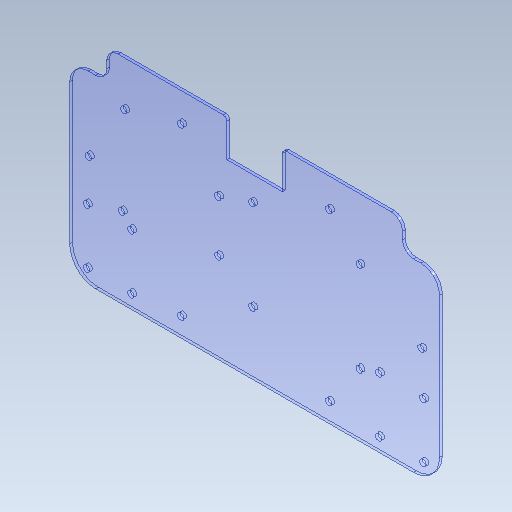
# Autodesk Inventor part: upper_frame
Saved by Autodesk Inventor 2020 (Build 240168000, 168)
## iProperties
Created: 2020-06-24
Part Number: upper_frame
Material: アルミニウム 6061
Document SubType Name: Modeling
Designer: haya
Density: 2.7 g/cm^3
Appearance: クリア - 青
Author: haya
Autodesk Inventor part; units mm, degrees
ref_plane "YZ Plane" through (0, 0, 0) normal (1, 0, 0) x (0, 1, 0)
ref_plane "XZ Plane" through (0, 0, 0) normal (0, 1, 0) x (-1, 0, 0)
ref_plane "XY Plane" through (0, 0, 0) normal (0, 0, 1) x (1, 0, 0)
sketch "スケッチ1" plane through (0, 0, 0) normal (0, 0, 1) x (1, 0, 0)
  line L0 (0, 0) -> (200, 0)
  line L1 (200, 0) -> (200, 100)
  line L2 (200, 100) -> (0, 100)
  line L3 (0, 100) -> (0, 0)
  dimension "d2" = 200
  dimension "d3" = 100
  constraints: 8 end point, 2 parallel, 1 horizontal, 1 perpendicular
  measures "d2" distance of L0.start L0.end
  measures "d3" distance of L2.end L0.start
extrude "押し出し1" add sketch "スケッチ1" along normal blind 1.5
fillet "フィレット1" radius 10 2 edges at (0, 100, 0.75) (200, 100, 0.75)
fillet "フィレット2" radius 14 2 edges at (200, 0, 0.75) (0, 0, 0.75)
sketch "スケッチ2" plane through (0, 0, 0) normal (0, 0, -1) x (-1, 0, 0)
  line L0 (-190, 100) -> (-10, 100) projected
  line L1 (-180, 100) -> (-20, 100)
  line L2 (-20, 100) -> (-20, 116)
  line L3 (-20, 116) -> (-180, 116)
  line L4 (-180, 116) -> (-180, 100)
  line L5 (0, 90) -> (0, 14) projected
  line L6 (-200, 14) -> (-200, 90) projected
  point P0 (0, 0)
  dimension "d6" = 20
  dimension "d7" = 20
  dimension "d8" = 16
  constraints: 8 end point, 2 parallel, 1 horizontal, 1 perpendicular, 1 point on line
  measures "d6" distance between parallel lines of L2 L5
  measures "d7" distance between parallel lines of L4 L6
  measures "d8" distance between parallel lines of L0 L3
extrude "押し出し2" add sketch "スケッチ2" against normal blind 1.5
fillet "フィレット3" radius 6 4 edges at (20, 100, 0.75) (20, 116, 0.75) (180, 116, 0.75) (180, 100, 0.75)
sketch "スケッチ3" plane through (0, 0, 0) normal (0, 0, -1) x (-1, 0, 0)
  line L0 (-14, 0) -> (-186, 0) projected
  line L1 (-200, 14) -> (-200, 90) projected
  line L2 (0, 90) -> (0, 14) projected
  point P0 (0, 0)
  point P1 (-167, 7)
  point P2 (-167, 37)
  point P3 (-191, 37)
  point P4 (-191, 7)
  point P5 (-9, 7)
  point P6 (-33, 7)
  point P7 (-9, 37)
  point P8 (-33, 37)
  dimension "d12" = 7
  dimension "d13" = 7
  dimension "d14" = 9
  dimension "d15" = 9
  dimension "d16" = 30
  dimension "d17" = 24
  dimension "d18" = 24
  dimension "d19" = 30
  dimension "d27" = 7
  dimension "d28" = 9
  dimension "d31" = 24
  dimension "d34" = 30
  constraints: 1 horizontal, 1 vertical, 3 other
  measures "d12" distance from line of point (-191, 7) L0
  measures "d13" distance from line of L0 point (-167, 7)
  measures "d14" distance from line of L1 point (-191, 7)
  measures "d15" distance from line of point (-191, 37) L1
  measures "d16" distance of point (-191, 37) point (-191, 7)
  measures "d17" distance of point (-167, 7) point (-191, 7)
  measures "d18" distance of point (-167, 37) point (-191, 37)
  measures "d19" distance of point (-167, 37) point (-167, 7)
  measures "d27" distance from line of point (-9, 7) L0
  measures "d28" distance from line of point (-9, 7) L2
  measures "d31" distance of point (-9, 7) point (-33, 7)
  measures "d34" distance of point (-9, 7) point (-9, 37)
hole "穴1" at (167, 7, 0) at (167, 37, 0) at (191, 37, 0) at (191, 7, 0) at (9, 7, 0) at (9, 37, 0) at (33, 37, 0) at (33, 7, 0) direction (0, 0, 1) diameter 3.5 end through all
sketch "スケッチ4" plane through (0, 0, 1.5) normal (0, 0, 1) x (1, 0, 0)
  line L0 (174, 116) -> (26, 116) projected
  line L1 (85, 116) -> (115, 116)
  line L2 (115, 116) -> (115, 96)
  line L3 (115, 96) -> (85, 96)
  line L4 (85, 96) -> (85, 116)
  line L5 (100, 116) -> (100, 0)
  line L6 (14, 0) -> (186, 0) projected
  point P0 (0, 0)
  dimension "d37" = 30
  dimension "d38" = 20
  constraints: 10 end point, 2 midpoint, 2 parallel, 1 horizontal, 1 perpendicular, 1 point on line, 1 other
  measures "d37" distance between parallel lines of L2 L4
  measures "d38" distance between parallel lines of L3 L0
extrude "押し出し3" cut sketch "スケッチ4" against normal through all
fillet "フィレット4" radius 2 2 edges at (85, 116, 0.75) (115, 116, 0.75)
sketch "スケッチ5" plane through (0, 0, 1.5) normal (0, 0, 1) x (1, 0, 0)
  circle A0 centre (10, 60) radius 1.5 projected
  circle A1 centre (60, 100) radius 1.5 projected
  circle A2 centre (60, 10) radius 1.5 projected
  circle A3 centre (140, 10) radius 1.5 projected
  circle A4 centre (190, 60) radius 1.5 projected
  circle A5 centre (140, 100) radius 1.5 projected
  point P0 (0, 0)
hole "穴2" at (60, 10, 1.5) at (10, 60, 1.5) at (60, 100, 1.5) at (140, 100, 1.5) at (190, 60, 1.5) at (140, 10, 1.5) direction (0, 0, -1) diameter 3.5 end through all
sketch "スケッチ6" plane through (0, 0, 1.5) normal (0, 0, 1) x (1, 0, 0)
  line L0 (14, 40.66) -> (80.04, 40.66) projected
  line L1 (14, 94) -> (14, 40.66) projected
  line L2 (80.04, 94) -> (14, 94) projected
  line L3 (80.04, 81.046) -> (80.04, 94) projected
  line L4 (82.58, 78.506) -> (80.04, 81.046) projected
  line L5 (82.58, 45.74) -> (82.58, 78.506) projected
  line L6 (80.04, 43.2) -> (82.58, 45.74) projected
  line L7 (80.04, 40.66) -> (80.04, 43.2) projected
  circle A0 centre (47.02, 43.2) radius 0.4 projected
  circle A1 centre (49.56, 43.2) radius 0.4 projected
  circle A2 centre (52.1, 43.2) radius 0.4 projected
  circle A3 centre (54.64, 43.2) radius 0.4 projected
  circle A4 centre (57.18, 43.2) radius 0.4 projected
  circle A5 centre (59.72, 43.2) radius 0.4 projected
  circle A6 centre (64.8, 43.2) radius 0.4 projected
  circle A7 centre (67.34, 43.2) radius 0.4 projected
  circle A8 centre (69.88, 43.2) radius 0.4 projected
  circle A9 centre (72.42, 43.2) radius 0.4 projected
  circle A10 centre (74.96, 43.2) radius 0.4 projected
  circle A11 centre (77.5, 43.2) radius 0.4 projected
  circle A12 centre (37.876, 91.46) radius 0.4 projected
  circle A13 centre (40.416, 91.46) radius 0.4 projected
  circle A14 centre (42.956, 91.46) radius 0.4 projected
  circle A15 centre (45.496, 91.46) radius 0.4 projected
  circle A16 centre (48.036, 91.46) radius 0.4 projected
  circle A17 centre (50.576, 91.46) radius 0.4 projected
  circle A18 centre (53.116, 91.46) radius 0.4 projected
  circle A19 centre (55.656, 91.46) radius 0.4 projected
  circle A20 centre (64.8, 91.46) radius 0.4 projected
  circle A21 centre (67.34, 91.46) radius 0.4 projected
  circle A22 centre (69.88, 91.46) radius 0.4 projected
  circle A23 centre (72.42, 91.46) radius 0.4 projected
  circle A24 centre (74.96, 91.46) radius 0.4 projected
  circle A25 centre (77.5, 91.46) radius 0.4 projected
  circle A26 centre (76.865, 53.233) radius 0.4 projected
  circle A27 centre (76.865, 60.853) radius 0.4 projected
  circle A28 centre (74.325, 53.233) radius 0.4 projected
  circle A29 centre (74.325, 60.853) radius 0.4 projected
  circle A30 centre (71.785, 53.233) radius 0.4 projected
  circle A31 centre (71.785, 60.853) radius 0.4 projected
  circle A32 centre (69.245, 53.233) radius 0.4 projected
  circle A33 centre (69.245, 60.853) radius 0.4 projected
  circle A34 centre (66.705, 53.233) radius 0.4 projected
  circle A35 centre (66.705, 60.853) radius 0.4 projected
  circle A36 centre (64.165, 53.233) radius 0.4 projected
  circle A37 centre (64.165, 60.853) radius 0.4 projected
  circle A38 centre (61.625, 53.233) radius 0.4 projected
  circle A39 centre (61.625, 60.853) radius 0.4 projected
  circle A40 centre (59.085, 53.233) radius 0.4 projected
  circle A41 centre (59.085, 60.853) radius 0.4 projected
  circle A42 centre (56.545, 53.233) radius 0.4 projected
  circle A43 centre (56.545, 60.853) radius 0.4 projected
  circle A44 centre (54.005, 53.233) radius 0.4 projected
  circle A45 centre (54.005, 60.853) radius 0.4 projected
  circle A46 centre (51.465, 53.233) radius 0.4 projected
  circle A47 centre (51.465, 60.853) radius 0.4 projected
  circle A48 centre (48.925, 53.233) radius 0.4 projected
  circle A49 centre (48.925, 60.853) radius 0.4 projected
  circle A50 centre (46.385, 53.233) radius 0.4 projected
  circle A51 centre (46.385, 60.853) radius 0.4 projected
  circle A52 centre (43.845, 53.233) radius 0.4 projected
  circle A53 centre (43.845, 60.853) radius 0.4 projected
  circle A54 centre (30.383, 66.822) radius 0.5 projected
  circle A55 centre (35.463, 66.822) radius 0.5 projected
  circle A56 centre (32.288, 80.538) radius 0.4 projected
  circle A57 centre (34.828, 80.538) radius 0.4 projected
  circle A58 centre (34.828, 83.078) radius 0.4 projected
  circle A59 centre (32.288, 83.078) radius 0.4 projected
  circle A60 centre (29.748, 85.618) radius 0.4 projected
  circle A61 centre (32.288, 85.618) radius 0.4 projected
  circle A62 centre (34.828, 85.618) radius 0.4 projected
  circle A63 centre (34.828, 88.158) radius 0.4 projected
  circle A64 centre (32.288, 88.158) radius 0.4 projected
  circle A65 centre (29.748, 88.158) radius 0.4 projected
  circle A66 centre (77.64, 71.09) radius 0.4 projected
  circle A67 centre (77.64, 68.55) radius 0.4 projected
  circle A68 centre (77.64, 66.01) radius 0.4 projected
  circle A69 centre (80.18, 66.01) radius 0.4 projected
  circle A70 centre (80.18, 68.55) radius 0.4 projected
  circle A71 centre (80.18, 71.09) radius 0.4 projected
  circle A72 centre (62.26, 91.46) radius 0.4 projected
  circle A73 centre (35.336, 91.46) radius 0.4 projected
  circle A74 centre (59.72, 91.46) radius 0.4 projected
  circle A75 centre (44.48, 43.2) radius 0.4 projected
  circle A76 centre (32.796, 91.46) radius 0.4 projected
  circle A77 centre (41.94, 43.2) radius 0.4 projected
  circle A78 centre (29.24, 91.46) radius 1.5875 projected
  circle A79 centre (27.97, 43.2) radius 1.5875 projected
  circle A80 centre (80.04, 76.22) radius 1.5875 projected
  circle A81 centre (80.04, 48.28) radius 1.5875 projected
  point P0 (0, 0)
hole "穴3" at (29.24, 91.46, 1.5) at (27.97, 43.2, 1.5) at (80.04, 48.28, 1.5) at (80.04, 76.22, 1.5) direction (0, 0, -1) diameter 3.5 end through all
sketch "スケッチ7" plane through (0, 0, 1.5) normal (0, 0, 1) x (1, 0, 0)
  line L0 (177, 86) -> (98, 86) projected
  arc A0 (180, 83) -> (177, 86) centre (177, 83) ccw projected
  line L1 (180, 33) -> (180, 83) projected
  arc A1 (177, 30) -> (180, 33) centre (177, 33) ccw projected
  line L2 (98, 30) -> (177, 30) projected
  arc A2 (95, 33) -> (98, 30) centre (98, 33) ccw projected
  line L3 (95, 83) -> (95, 33) projected
  arc A3 (98, 86) -> (95, 83) centre (98, 83) ccw projected
  circle A4 centre (98.5, 33.5) radius 3 projected
  circle A5 centre (156.5, 33.5) radius 3 projected
  circle A6 centre (157.77, 75.09) radius 0.5 projected
  circle A7 centre (155.23, 75.09) radius 0.5 projected
  circle A8 centre (108.45, 83.77) radius 0.5 projected
  circle A9 centre (110.99, 83.77) radius 0.5 projected
  circle A10 centre (113.53, 83.77) radius 0.5 projected
  circle A11 centre (116.07, 83.77) radius 0.5 projected
  circle A12 centre (118.61, 83.77) radius 0.5 projected
  circle A13 centre (121.15, 83.77) radius 0.5 projected
  circle A14 centre (123.69, 83.77) radius 0.5 projected
  circle A15 centre (126.23, 83.77) radius 0.5 projected
  circle A16 centre (128.77, 83.77) radius 0.5 projected
  circle A17 centre (131.31, 83.77) radius 0.5 projected
  circle A18 centre (133.85, 83.77) radius 0.5 projected
  circle A19 centre (136.39, 83.77) radius 0.5 projected
  circle A20 centre (138.93, 83.77) radius 0.5 projected
  circle A21 centre (141.47, 83.77) radius 0.5 projected
  circle A22 centre (144.01, 83.77) radius 0.5 projected
  circle A23 centre (146.55, 83.77) radius 0.5 projected
  circle A24 centre (149.09, 83.77) radius 0.5 projected
  circle A25 centre (151.63, 83.77) radius 0.5 projected
  circle A26 centre (103.37, 81.23) radius 0.5 projected
  circle A27 centre (105.91, 81.23) radius 0.5 projected
  circle A28 centre (108.45, 81.23) radius 0.5 projected
  circle A29 centre (110.99, 81.23) radius 0.5 projected
  circle A30 centre (113.53, 81.23) radius 0.5 projected
  circle A31 centre (116.07, 81.23) radius 0.5 projected
  circle A32 centre (118.61, 81.23) radius 0.5 projected
  circle A33 centre (121.15, 81.23) radius 0.5 projected
  circle A34 centre (123.69, 81.23) radius 0.5 projected
  circle A35 centre (126.23, 81.23) radius 0.5 projected
  circle A36 centre (128.77, 81.23) radius 0.5 projected
  circle A37 centre (131.31, 81.23) radius 0.5 projected
  circle A38 centre (133.85, 81.23) radius 0.5 projected
  circle A39 centre (136.39, 81.23) radius 0.5 projected
  circle A40 centre (138.93, 81.23) radius 0.5 projected
  circle A41 centre (141.47, 81.23) radius 0.5 projected
  circle A42 centre (144.01, 81.23) radius 0.5 projected
  circle A43 centre (146.55, 81.23) radius 0.5 projected
  circle A44 centre (149.09, 81.23) radius 0.5 projected
  circle A45 centre (151.63, 81.23) radius 0.5 projected
  circle A46 centre (109.5, 50.5) radius 0.5 projected
  circle A47 centre (104.5, 50.5) radius 0.5 projected
  circle A48 centre (107, 50.5) radius 0.5 projected
  circle A49 centre (105.91, 83.77) radius 0.5 projected
  circle A50 centre (103.37, 83.77) radius 0.5 projected
  circle A51 centre (155.23, 77.63) radius 0.5 projected
  circle A52 centre (157.77, 77.63) radius 0.5 projected
  circle A53 centre (156.5, 82.5) radius 3 projected
  circle A54 centre (98.5, 82.5) radius 3 projected
  point P0 (0, 0)
hole "穴4" at (156.5, 33.5, 1.5) at (98.5, 33.5, 1.5) at (98.5, 82.5, 1.5) at (156.5, 82.5, 1.5) direction (0, 0, -1) diameter 3.5 end through all
